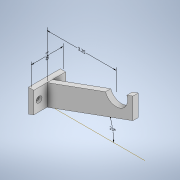
# Autodesk Inventor part: irrigationPipeSupport02
Saved by Autodesk Inventor 2021.1 (Build 251245010, 245A)
## iProperties
Created: 2020-09-15
Part Number: irrigationPipeSupport02
Material: Generic
Document SubType Name: Modeling
Designer: robst
Density: 1 g/cm^3
Appearance: Default
Author: robst
Autodesk Inventor part; units mm, degrees
ref_plane "YZ Plane" through (0, 0, 0) normal (1, 0, 0) x (0, 1, 0)
ref_plane "XZ Plane" through (0, 0, 0) normal (0, 1, 0) x (-1, 0, 0)
ref_plane "XY Plane" through (0, 0, 0) normal (0, 0, 1) x (1, 0, 0)
sketch "Sketch5" plane through (0, 0, 0) normal (0, 0, 1) x (1, 0, 0)
  line L0 (0, 0) -> (6.35, 0)
  line L1 (6.35, 0) -> (6.35, 25.4)
  line L2 (6.35, 25.4) -> (0, 25.4)
  line L3 (0, 25.4) -> (0, 0)
  dimension "d21" = 25.4
  dimension "d22" = 6.35
  constraints: 8 end point, 2 parallel, 1 horizontal, 1 perpendicular
  measures "d21" distance from line of L2 L0.start
  measures "d22" distance from line of L1 L0.start
extrude "Extrusion3" add sketch "Sketch5" against normal mid plane 38.1
sketch "Sketch6" plane through (0, 0, 0) normal (0, 0, 1) x (1, 0, 0)
  line L0 (6.35, 25.4) -> (6.35, 0) projected
  line L1 (0, 25.4) -> (6.35, 25.4) projected
  line L2 (6.35, 0) -> (0, 0) projected
  line L3 (0, 0) -> (0, 25.4) projected
  line L4 (6.35, 0) -> (108.9025, 37.3261)
  line L5 (6.35, 0) -> (115.4841, 0) construction
  line L6 (108.9025, 62.7261) -> (108.9025, 37.3261)
  arc A0 (76.0708, 50.7763) -> (101.7292, 60.1152) centre (88.9, 55.4457) ccw
  line L7 (6.35, 25.4) -> (76.0708, 50.7763)
  line L8 (101.7292, 60.1152) -> (108.9025, 62.7261)
  dimension "d25" = 20
  dimension "d26" = 27.305
  dimension "d29" = 6.35
  dimension "d30" = 88.9
  dimension "d33" = 0
  constraints: 10 end point, 2 parallel, 2 point on circle, 1 centre point, 1 collinear, 1 equal length, 1 horizontal, 1 vertical
  measures "d25" angle of L5 L4
  measures "d26" diameter of A0
  measures "d29" distance edge to line of A0 L6
  measures "d30" distance from line of A0.centre L3
  measures "d33" distance from line of L7 A0.centre
extrude "Extrusion4" add sketch "Sketch6" along normal mid plane 6.35 contours L7 A0 L8 L6 L4 L0
sketch "Sketch7" plane through (6.35, 0, 19.05) normal (1, 0, 0) x (0, 0, -1)
  line L0 (38.1, 25.4) -> (0, 25.4) construction
  line L1 (6.35, 25.4) -> (6.35, 0) construction
  line L2 (31.75, 25.4) -> (31.75, 0) construction
  line L3 (0, 0) -> (0, 25.4) construction
  line L4 (38.1, 25.4) -> (38.1, 0) construction
  line L5 (0, 0) -> (15.875, 0) projected
  line L6 (22.225, 0) -> (38.1, 0) projected
  point P0 (19.05, 0)
  point P1 (6.35, 12.7)
  point P2 (31.75, 12.7)
  dimension "d34" = 6.35
  dimension "d35" = 6.35
  constraints: 4 end point, 2 midpoint, 2 point on line, 2 vertical
  measures "d34" distance between parallel lines of L1 L3
  measures "d35" distance between parallel lines of L2 L4
sketch "Sketch8" plane through (0, 0, 0) normal (0, 0, 1) x (1, 0, 0)
  line L0 (0, 0) -> (0, 25.4) projected
  line L1 (6.35, 0) -> (0, 0) projected
  line L2 (108.9025, 37.3261) -> (6.35, 0) projected
  line L3 (0, 0) -> (6.35, 0)
  line L4 (0, -2.3112) -> (6.35, 0)
  line L5 (0, 0) -> (0, -2.3112)
  constraints: 6 end point, 2 collinear, 1 vertical
extrude "Extrusion5" add sketch "Sketch8" along normal mid plane 38.1
hole "Hole3" at (6.35, 12.7, 12.7) at (6.35, 12.7, -12.7) direction (-1, 0, 0) diameter 3.81 end through all countersink diameter 7.0866 countersink angle 82 clearance for "Flat Head Machine Screw (82)" size "#6" standard "Ansi Unified Screw Threads"
sketch "Sketch9" plane through (0, 25.4, -19.05) normal (-1, 0, 0) x (0, 0, 1)
  line L0 (0, -27.7112) -> (0, 0) projected
  line L1 (38.1, 0) -> (38.1, -27.7112) projected
  line L2 (0, -13.8556) -> (38.1, -13.8556) construction
  spline S0 degree 2 poles (10.605, -12.6206) (10.4939, -12.6206) (10.274, -12.6749) (10.1678, -12.7169) knots 0 0 0 1 2 2 2
  spline S1 degree 2 poles (10.1678, -12.7169) (10.069, -12.7589) (9.9233, -12.8478) (9.8665, -12.8874) knots 0 0 0 1 2 2 2
  line L3 (9.8665, -12.8874) -> (9.8418, -12.8874)
  line L4 (9.8418, -12.8874) -> (9.8418, -12.4551)
  spline S2 degree 2 poles (9.8418, -12.4551) (9.9752, -12.3835) (10.4321, -12.2674) (10.6371, -12.2674) knots 0 0 0 1 2 2 2
  spline S3 degree 2 poles (10.6371, -12.2674) (10.8446, -12.2674) (11.1534, -12.3514) (11.2793, -12.4403) knots 0 0 0 1 2 2 2
  spline S4 degree 2 poles (11.2793, -12.4403) (11.4127, -12.5366) (11.551, -12.8157) (11.551, -13.0034) knots 0 0 0 1 2 2 2
  spline S5 degree 2 poles (11.551, -13.0034) (11.551, -13.2554) (11.22, -13.6358) (10.9879, -13.6852) knots 0 0 0 1 2 2 2
  line L5 (10.9879, -13.6852) -> (10.9879, -13.7148)
  spline S6 degree 2 poles (10.9879, -13.7148) (11.0842, -13.7346) (11.304, -13.8235) (11.3979, -13.9124) knots 0 0 0 1 2 2 2
  spline S7 degree 2 poles (11.3979, -13.9124) (11.4918, -13.9989) (11.6103, -14.2755) (11.6103, -14.4756) knots 0 0 0 1 2 2 2
  spline S8 degree 2 poles (11.6103, -14.4756) (11.6103, -14.6806) (11.4695, -15.0289) (11.3411, -15.1622) knots 0 0 0 1 2 2 2
  spline S9 degree 2 poles (11.3411, -15.1622) (11.2077, -15.3006) (10.8298, -15.4438) (10.5902, -15.4438) knots 0 0 0 1 2 2 2
  spline S10 degree 2 poles (10.5902, -15.4438) (10.3605, -15.4438) (9.9109, -15.3327) (9.7578, -15.2561) knots 0 0 0 1 2 2 2
  line L6 (9.7578, -15.2561) -> (9.7578, -14.8239)
  line L7 (9.7578, -14.8239) -> (9.7874, -14.8239)
  spline S11 degree 2 poles (9.7874, -14.8239) (9.9159, -14.9177) (10.3506, -15.0906) (10.5655, -15.0906) knots 0 0 0 1 2 2 2
  spline S12 degree 2 poles (10.5655, -15.0906) (10.6915, -15.0906) (10.9434, -15.0116) (11.0274, -14.9202) knots 0 0 0 1 2 2 2
  spline S13 degree 2 poles (11.0274, -14.9202) (11.1089, -14.8288) (11.1953, -14.6114) (11.1953, -14.4459) knots 0 0 0 1 2 2 2
  spline S14 degree 2 poles (11.1953, -14.4459) (11.1953, -14.2804) (11.099, -14.0656) (11.0126, -14.0038) knots 0 0 0 1 2 2 2
  spline S15 degree 2 poles (11.0126, -14.0038) (10.9261, -13.9421) (10.6915, -13.8951) (10.5531, -13.8951) knots 0 0 0 1 2 2 2
  line L8 (10.5531, -13.8951) -> (10.3802, -13.8951)
  line L9 (10.3802, -13.8951) -> (10.3802, -13.5567)
  line L10 (10.3802, -13.5567) -> (10.5161, -13.5567)
  spline S16 degree 2 poles (10.5161, -13.5567) (10.7903, -13.5567) (11.1361, -13.2949) (11.1361, -13.0454) knots 0 0 0 1 2 2 2
  spline S17 degree 2 poles (11.1361, -13.0454) (11.1361, -12.9293) (11.0471, -12.7639) (10.9755, -12.7145) knots 0 0 0 1 2 2 2
  spline S18 degree 2 poles (10.9755, -12.7145) (10.8989, -12.6626) (10.7112, -12.6206) (10.605, -12.6206) knots 0 0 0 1 2 2 2
  line L11 (12.7243, -15.3796) -> (12.2352, -15.3796)
  line L12 (12.2352, -15.3796) -> (12.2352, -14.7967)
  line L13 (12.2352, -14.7967) -> (12.7243, -14.7967)
  line L14 (12.7243, -14.7967) -> (12.7243, -15.3796)
  line L15 (15.219, -15.3796) -> (13.3393, -15.3796)
  line L16 (13.3393, -15.3796) -> (13.3393, -14.9474)
  spline S19 degree 2 poles (13.3393, -14.9474) (13.5419, -14.7572) (13.9025, -14.4039) (14.0754, -14.2138) knots 0 0 0 1 2 2 2
  spline S20 degree 2 poles (14.0754, -14.2138) (14.4237, -13.8309) (14.6781, -13.3715) (14.6781, -13.127) knots 0 0 0 1 2 2 2
  spline S21 degree 2 poles (14.6781, -13.127) (14.6781, -12.9985) (14.599, -12.8058) (14.5274, -12.7441) knots 0 0 0 1 2 2 2
  spline S22 degree 2 poles (14.5274, -12.7441) (14.4558, -12.6823) (14.268, -12.6206) (14.1544, -12.6206) knots 0 0 0 1 2 2 2
  spline S23 degree 2 poles (14.1544, -12.6206) (14.0457, -12.6206) (13.8234, -12.6749) (13.7222, -12.7169) knots 0 0 0 1 2 2 2
  spline S24 degree 2 poles (13.7222, -12.7169) (13.6357, -12.7515) (13.4752, -12.8503) (13.4258, -12.8849) knots 0 0 0 1 2 2 2
  line L17 (13.4258, -12.8849) -> (13.4035, -12.8849)
  line L18 (13.4035, -12.8849) -> (13.4035, -12.4502)
  spline S25 degree 2 poles (13.4035, -12.4502) (13.5295, -12.3884) (13.9815, -12.2674) (14.1841, -12.2674) knots 0 0 0 1 2 2 2
  spline S26 degree 2 poles (14.1841, -12.2674) (14.6114, -12.2674) (15.093, -12.7194) (15.093, -13.1047) knots 0 0 0 1 2 2 2
  spline S27 degree 2 poles (15.093, -13.1047) (15.093, -13.285) (15.0091, -13.5864) (14.935, -13.7148) knots 0 0 0 1 2 2 2
  spline S28 degree 2 poles (14.935, -13.7148) (14.8609, -13.8482) (14.646, -14.11) (14.5274, -14.236) knots 0 0 0 1 2 2 2
  spline S29 degree 2 poles (14.5274, -14.236) (14.3347, -14.4459) (13.863, -14.8955) (13.7222, -15.0264) knots 0 0 0 1 2 2 2
  line L19 (13.7222, -15.0264) -> (15.219, -15.0264)
  line L20 (15.219, -15.0264) -> (15.219, -15.3796)
  spline S30 degree 2 poles (17.4741, -14.4114) (17.4741, -14.6312) (17.3333, -15.0066) (17.2049, -15.145) knots 0 0 0 1 2 2 2
  spline S31 degree 2 poles (17.2049, -15.145) (17.0765, -15.2833) (16.6936, -15.4438) (16.4565, -15.4438) knots 0 0 0 1 2 2 2
  spline S32 degree 2 poles (16.4565, -15.4438) (16.2391, -15.4438) (15.8143, -15.3475) (15.6587, -15.2709) knots 0 0 0 1 2 2 2
  line L21 (15.6587, -15.2709) -> (15.6587, -14.8387)
  line L22 (15.6587, -14.8387) -> (15.6883, -14.8387)
  spline S33 degree 2 poles (15.6883, -14.8387) (15.7352, -14.8733) (15.9106, -14.9622) (16.0168, -15.0017) knots 0 0 0 1 2 2 2
  spline S34 degree 2 poles (16.0168, -15.0017) (16.1379, -15.0437) (16.3379, -15.0906) (16.4639, -15.0906) knots 0 0 0 1 2 2 2
  spline S35 degree 2 poles (16.4639, -15.0906) (16.5874, -15.0906) (16.8196, -15.0017) (16.9036, -14.9054) knots 0 0 0 1 2 2 2
  spline S36 degree 2 poles (16.9036, -14.9054) (16.9801, -14.814) (17.0592, -14.5719) (17.0592, -14.4089) knots 0 0 0 1 2 2 2
  spline S37 degree 2 poles (17.0592, -14.4089) (17.0592, -14.2459) (16.9702, -14.0384) (16.8863, -13.9692) knots 0 0 0 1 2 2 2
  spline S38 degree 2 poles (16.8863, -13.9692) (16.7998, -13.8927) (16.5429, -13.8284) (16.3873, -13.8284) knots 0 0 0 1 2 2 2
  spline S39 degree 2 poles (16.3873, -13.8284) (16.2194, -13.8284) (15.8859, -13.8803) (15.7846, -13.9025) knots 0 0 0 1 2 2 2
  line L23 (15.7846, -13.9025) -> (15.7846, -12.3316)
  line L24 (15.7846, -12.3316) -> (17.4568, -12.3316)
  line L25 (17.4568, -12.3316) -> (17.4568, -12.6898)
  line L26 (17.4568, -12.6898) -> (16.1774, -12.6898)
  line L27 (16.1774, -12.6898) -> (16.1774, -13.5024)
  spline S40 degree 2 poles (16.1774, -13.5024) (16.2515, -13.4925) (16.3947, -13.4851) (16.454, -13.4851) knots 0 0 0 1 2 2 2
  spline S41 degree 2 poles (16.454, -13.4851) (16.6887, -13.4851) (17.0122, -13.5617) (17.1604, -13.6753) knots 0 0 0 1 2 2 2
  spline S42 degree 2 poles (17.1604, -13.6753) (17.3111, -13.7889) (17.4741, -14.1347) (17.4741, -14.4114) knots 0 0 0 1 2 2 2
  line L28 (18.3707, -12.1958) -> (18.2818, -13.3814)
  line L29 (18.2818, -13.3814) -> (18.0126, -13.3814)
  line L30 (18.0126, -13.3814) -> (17.9237, -12.1958)
  line L31 (17.9237, -12.1958) -> (18.3707, -12.1958)
  line L32 (19.1414, -12.1958) -> (19.0525, -13.3814)
  line L33 (19.0525, -13.3814) -> (18.7832, -13.3814)
  line L34 (18.7832, -13.3814) -> (18.6943, -12.1958)
  line L35 (18.6943, -12.1958) -> (19.1414, -12.1958)
  line L36 (22.7847, -15.3796) -> (20.905, -15.3796)
  line L37 (20.905, -15.3796) -> (20.905, -14.9474)
  spline S43 degree 2 poles (20.905, -14.9474) (21.1075, -14.7572) (21.4681, -14.4039) (21.641, -14.2138) knots 0 0 0 1 2 2 2
  spline S44 degree 2 poles (21.641, -14.2138) (21.9893, -13.8309) (22.2437, -13.3715) (22.2437, -13.127) knots 0 0 0 1 2 2 2
  spline S45 degree 2 poles (22.2437, -13.127) (22.2437, -12.9985) (22.1647, -12.8058) (22.0931, -12.7441) knots 0 0 0 1 2 2 2
  spline S46 degree 2 poles (22.0931, -12.7441) (22.0214, -12.6823) (21.8337, -12.6206) (21.7201, -12.6206) knots 0 0 0 1 2 2 2
  spline S47 degree 2 poles (21.7201, -12.6206) (21.6114, -12.6206) (21.3891, -12.6749) (21.2878, -12.7169) knots 0 0 0 1 2 2 2
  spline S48 degree 2 poles (21.2878, -12.7169) (21.2014, -12.7515) (21.0408, -12.8503) (20.9914, -12.8849) knots 0 0 0 1 2 2 2
  line L38 (20.9914, -12.8849) -> (20.9692, -12.8849)
  line L39 (20.9692, -12.8849) -> (20.9692, -12.4502)
  spline S49 degree 2 poles (20.9692, -12.4502) (21.0952, -12.3884) (21.5472, -12.2674) (21.7497, -12.2674) knots 0 0 0 1 2 2 2
  spline S50 degree 2 poles (21.7497, -12.2674) (22.177, -12.2674) (22.6587, -12.7194) (22.6587, -13.1047) knots 0 0 0 1 2 2 2
  spline S51 degree 2 poles (22.6587, -13.1047) (22.6587, -13.285) (22.5747, -13.5864) (22.5006, -13.7148) knots 0 0 0 1 2 2 2
  spline S52 degree 2 poles (22.5006, -13.7148) (22.4265, -13.8482) (22.2116, -14.11) (22.0931, -14.236) knots 0 0 0 1 2 2 2
  spline S53 degree 2 poles (22.0931, -14.236) (21.9004, -14.4459) (21.4286, -14.8955) (21.2878, -15.0264) knots 0 0 0 1 2 2 2
  line L40 (21.2878, -15.0264) -> (22.7847, -15.0264)
  line L41 (22.7847, -15.0264) -> (22.7847, -15.3796)
  spline S54 degree 2 poles (25.0892, -13.8556) (25.0892, -14.6757) (24.6125, -15.4438) (24.116, -15.4438) knots 0 0 0 1 2 2 2
  spline S55 degree 2 poles (24.116, -15.4438) (23.6121, -15.4438) (23.1403, -14.6608) (23.1403, -13.8581) knots 0 0 0 1 2 2 2
  spline S56 degree 2 poles (23.1403, -13.8581) (23.1403, -13.0331) (23.6171, -12.2699) (24.116, -12.2699) knots 0 0 0 1 2 2 2
  spline S57 degree 2 poles (24.116, -12.2699) (24.6174, -12.2699) (25.0892, -13.0603) (25.0892, -13.8556) knots 0 0 0 1 2 2 2
  spline S58 degree 2 poles (24.5655, -14.7843) (24.6248, -14.6337) (24.6742, -14.1693) (24.6742, -13.8556) knots 0 0 0 1 2 2 2
  spline S59 degree 2 poles (24.6742, -13.8556) (24.6742, -13.5419) (24.6248, -13.08) (24.5631, -12.9244) knots 0 0 0 1 2 2 2
  spline S60 degree 2 poles (24.5631, -12.9244) (24.5013, -12.7688) (24.2864, -12.6082) (24.116, -12.6082) knots 0 0 0 1 2 2 2
  spline S61 degree 2 poles (24.116, -12.6082) (23.9456, -12.6082) (23.7257, -12.7688) (23.6615, -12.9293) knots 0 0 0 1 2 2 2
  spline S62 degree 2 poles (23.6615, -12.9293) (23.5998, -13.085) (23.5553, -13.5592) (23.5553, -13.8581) knots 0 0 0 1 2 2 2
  spline S63 degree 2 poles (23.5553, -13.8581) (23.5553, -14.1792) (23.5948, -14.609) (23.6591, -14.7769) knots 0 0 0 1 2 2 2
  spline S64 degree 2 poles (23.6591, -14.7769) (23.7183, -14.935) (23.9382, -15.1054) (24.116, -15.1054) knots 0 0 0 1 2 2 2
  spline S65 degree 2 poles (24.116, -15.1054) (24.284, -15.1054) (24.5038, -14.9449) (24.5655, -14.7843) knots 0 0 0 1 2 2 2
  spline S66 degree 2 poles (27.0232, -13.0578) (27.0232, -13.3863) (26.5737, -13.8358) (26.2452, -13.8358) knots 0 0 0 1 2 2 2
  spline S67 degree 2 poles (26.2452, -13.8358) (25.9191, -13.8358) (25.4646, -13.3888) (25.4646, -13.0578) knots 0 0 0 1 2 2 2
  spline S68 degree 2 poles (25.4646, -13.0578) (25.4646, -12.7293) (25.9142, -12.2797) (26.2452, -12.2797) knots 0 0 0 1 2 2 2
  spline S69 degree 2 poles (26.2452, -12.2797) (26.5737, -12.2797) (27.0232, -12.7293) (27.0232, -13.0578) knots 0 0 0 1 2 2 2
  spline S70 degree 2 poles (26.7021, -13.0578) (26.7021, -12.8602) (26.4403, -12.591) (26.2452, -12.591) knots 0 0 0 1 2 2 2
  spline S71 degree 2 poles (26.2452, -12.591) (26.0476, -12.591) (25.7857, -12.8602) (25.7857, -13.0578) knots 0 0 0 1 2 2 2
  spline S72 degree 2 poles (25.7857, -13.0578) (25.7857, -13.2579) (26.0525, -13.5246) (26.2452, -13.5246) knots 0 0 0 1 2 2 2
  spline S73 degree 2 poles (26.2452, -13.5246) (26.4403, -13.5246) (26.7021, -13.2529) (26.7021, -13.0578) knots 0 0 0 1 2 2 2
  point P0 (19.05, -25.4)
  constraints: 2 end point, 2 midpoint, 1 horizontal
extrude "Extrusion6" cut sketch "Sketch9" against normal blind 1.27
equation "\"d21\" = supportHeight"
equation "\"d22\" = supportWidth"
equation "\"d23\" = totalScrewHoldWidth"
equation "\"d25\" = supportAngle"
equation "\"d26\" = pipeDiameter"
equation "\"d30\" = distanceFromWallToPipeCenter"
equation "\"d31\" = supportWidth"
equation "\"d47\" = totalScrewHoldWidth"
equation "\"pipeDiameter\" = 27.305"
equation "\"distanceFromWallToPipeCenter\" = 88.9"
equation "\"supportHeight\" = 25.4"
equation "\"supportWidth\" = 6.35"
equation "\"screwHoldDepth\" = 6.35"
equation "\"totalScrewHoldWidth\" = 38.1"
equation "\"screwPositionFromTop\" = 6.35"
equation "\"supportAngle\" = 20deg"
body "Solid1"
body "Solid2"
